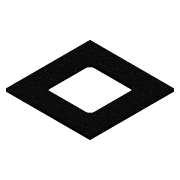
# Autodesk Inventor part: 00_ZEISS_Axiotech_Plate
Saved by Autodesk Inventor 2019 (Build 230136000, 136)
## iProperties
Created: 2019-05-02
Part Number: 00_ZEISS_Axiotech_Plate
Material: Generic
Document SubType Name: Modeling
Designer: diederichbenedict
Density: 1 g/cm^3
Appearance: Black
Author: diederichbenedict
Autodesk Inventor part; units mm, degrees
ref_plane "YZ Plane" through (0, 0, 0) normal (1, 0, 0) x (0, 1, 0)
ref_plane "XZ Plane" through (0, 0, 0) normal (0, 1, 0) x (-1, 0, 0)
ref_plane "XY Plane" through (0, 0, 0) normal (0, 0, 1) x (1, 0, 0)
sketch "Sketch1" plane through (0, 0, 0) normal (0, 1, 0) x (-1, 0, 0)
  line L0 (-65, -80) -> (65, -80)
  line L1 (80, -65) -> (80, 65)
  line L2 (65, 80) -> (-65, 80)
  line L3 (-80, 65) -> (-80, -65)
  line L4 (-80, -80) -> (80, 80) construction
  line L5 (80, -80) -> (-80, 80) construction
  arc A0 (80, 65) -> (65, 80) centre (65, 65) ccw
  arc A1 (-65, 80) -> (-80, 65) centre (-65, 65) ccw
  arc A2 (-80, -65) -> (-65, -80) centre (-65, -65) ccw
  arc A3 (65, -80) -> (80, -65) centre (65, -65) ccw
  line L6 (-150, -150) -> (150, -150)
  line L7 (150, -150) -> (150, 150)
  line L8 (150, 150) -> (-150, 150)
  line L9 (-150, 150) -> (-150, -150)
  line L10 (-150, -150) -> (150, 150) construction
  line L11 (150, -150) -> (-150, 150) construction
  point P0 (0, 0)
  dimension "d0" = 160
  dimension "d1" = 160
  dimension "d2" = 15
  dimension "d3" = 300
  dimension "d4" = 300
  constraints: 24 end point, 8 point on circle, 8 point on line, 8 tangent, 4 centre point, 4 midpoint, 4 parallel, 3 equal radius, 2 horizontal, 2 perpendicular
  measures "d0" distance of L5.end L4.end
  measures "d1" distance of L4.end L5.start
  measures "d2" radius of A0
  measures "d3" distance of L8.end L7.end
  measures "d4" distance of L7.end L6.end
extrude "Extrusion1" add sketch "Sketch1" along normal blind 10
sketch "Sketch2" plane through (0, 10, 0) normal (0, 1, 0) x (1, 0, 0)
  circle A0 centre (-67, -107.5) radius 1.95 projected
  circle A1 centre (67, -107.5) radius 1.95 projected
  circle A2 centre (67, 107.5) radius 1.95 projected
  circle A3 centre (-67, 107.5) radius 1.95 projected
  point P0 (0, 0)
extrude "Extrusion2" cut sketch "Sketch2" against normal blind 10
body "Solid1"
